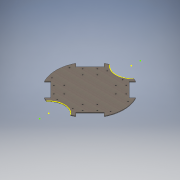
# Autodesk Inventor part: floor_v2
Saved by Autodesk Inventor 2020 (Build 240168000, 168)
## iProperties
Created: 2024-09-07
Part Number: floor_v2
Material: Алюминий 6061
Document SubType Name: Modeling
Designer: Ivan
Density: 2.7 g/cm^3
Appearance: Орех
Mass: 210.887 g
Surface Area: 551.998 cm^2
Volume: 78.1062 cm^3
Author: Ivan
Autodesk Inventor part; units mm, degrees
ref_plane "YZ Plane" through (0, 0, 0) normal (1, 0, 0) x (0, 1, 0)
ref_plane "XZ Plane" through (0, 0, 0) normal (0, 1, 0) x (-1, 0, 0)
ref_plane "XY Plane" through (0, 0, 0) normal (0, 0, 1) x (1, 0, 0)
sketch "Эскиз2" plane through (0, 0, 0) normal (0, 1, 0) x (1, 0, 0)
  circle A0 centre (0, 0) radius 107.5
  circle A1 centre (0, 0) radius 104
  line L0 (0, 0) -> (104, 0) construction
  line L1 (0, 0) -> (0, -104) construction
  line L2 (0, 0) -> (-104, 0) construction
  line L3 (0, 0) -> (0, 104) construction
  line L4 (104, 0) -> (0, -104) construction
  line L5 (0, 104) -> (-104, 0) construction
  line L6 (0, -104) -> (-104, 0) construction
  line L7 (104, 0) -> (0, 104) construction
  line L8 (0, 0) -> (-73.5391, -73.5391) construction
  line L9 (0, 0) -> (73.5391, -73.5391) construction
  line L10 (0, 0) -> (73.5391, 73.5391) construction
  line L11 (0, 0) -> (-73.5391, 73.5391) construction
  line L12 (-38.4471, -82.2877) -> (-82.2877, -38.4471)
  line L13 (-38.4471, -82.2877) -> (-48.2758, -92.1165)
  line L14 (-82.2877, -38.4471) -> (-92.1165, -48.2758)
  line L15 (92.1165, -48.2758) -> (82.2877, -38.4471)
  line L16 (82.2877, -38.4471) -> (38.4471, -82.2877)
  line L17 (38.4471, -82.2877) -> (48.2758, -92.1165)
  line L18 (48.2758, 92.1165) -> (38.4471, 82.2877)
  line L19 (38.4471, 82.2877) -> (82.2877, 38.4471)
  line L20 (82.2877, 38.4471) -> (92.1165, 48.2758)
  line L21 (-48.2758, 92.1165) -> (-38.4471, 82.2877)
  line L22 (-38.4471, 82.2877) -> (-82.2877, 38.4471)
  line L23 (-82.2877, 38.4471) -> (-92.1165, 48.2758)
  line L24 (0, -107.5) -> (0, -79.5) construction
  circle A2 centre (0, -116.5) radius 37 construction
  circle A3 centre (0, -127) radius 47.5
  line L25 (0, 107.5) -> (0, 79.5) construction
  circle A4 centre (0, 127) radius 47.5
  line L26 (-92.1165, 48.2758) -> (-94.7051, 50.8645)
  line L27 (-48.2758, 92.1165) -> (-50.8645, 94.7051)
  line L28 (48.2758, 92.1165) -> (50.8645, 94.7051)
  line L29 (92.1165, 48.2758) -> (94.7051, 50.8645)
  line L30 (92.1165, -48.2758) -> (94.7051, -50.8645)
  line L31 (48.2758, -92.1165) -> (50.8645, -94.7051)
  line L32 (-92.1165, -48.2758) -> (-94.7051, -50.8645)
  line L33 (-48.2758, -92.1165) -> (-50.8645, -94.7051)
  point P0 (-52, -52)
  point P1 (-52, 52)
  point P2 (52, 52)
  point P3 (52, -52)
  point P4 (-60.3674, -60.3674)
  point P5 (60.3674, -60.3674)
  point P6 (60.3674, 60.3674)
  point P7 (-60.3674, 60.3674)
  point P8 (-36.9892, -97.1998)
  point P9 (36.9892, -97.1998)
  point P10 (36.9892, 97.1998)
  point P11 (-36.9892, 97.1998)
  dimension "d137" = 215
  dimension "d138" = 208
  dimension "d143" = 74
  dimension "d144" = 95
  dimension "d140" = 62
  dimension "d141" = 13.9
  dimension "d142" = 28
  constraints: 68 end point, 15 point on line, 14 equal length, 10 perpendicular, 8 collinear, 8 midpoint, 5 parallel, 2 coincident, 2 horizontal, 2 vertical, 1 vertical alignment, 32 other
  measures "d140" distance from line of L14 L12.start
  measures "d141" distance from line of L12 L13.end
  measures "d142" distance of L24.start L24.end
extrude "Выдавливание1" add sketch "Эскиз2" along normal blind 2 contours A1 L15 L16 L17 A3 L13 L12 L14 L23 L22 L21 A4 L18 L19 L20
sketch "Эскиз3" plane through (0, 2, 0) normal (0, -1, 0) x (-1, 0, 0)
  line L0 (33.8509, 77.6915) -> (77.6915, 33.8509) construction
  line L1 (55.7712, 55.7712) -> (0, 0) construction
  line L2 (44.4575, 67.0849) -> (67.0849, 44.4575) construction
  circle A0 centre (44.4575, 67.0849) radius 1.5
  circle A1 centre (67.0849, 44.4575) radius 1.5
  line L3 (28.3991, 51.0265) -> (51.0265, 28.3991) construction
  circle A2 centre (28.3991, 51.0265) radius 1.5
  circle A3 centre (51.0265, 28.3991) radius 1.5
  line L4 (44.4575, -67.0849) -> (67.0849, -44.4575) construction
  line L5 (28.3991, -51.0265) -> (51.0265, -28.3991) construction
  line L6 (55.7712, -55.7712) -> (0, 0) construction
  line L7 (-44.4575, -67.0849) -> (-67.0849, -44.4575) construction
  line L8 (-28.3991, -51.0265) -> (-51.0265, -28.3991) construction
  line L9 (-55.7712, -55.7712) -> (0, 0) construction
  line L10 (-67.0849, 44.4575) -> (-44.4575, 67.0849) construction
  line L11 (-51.0265, 28.3991) -> (-28.3991, 51.0265) construction
  line L12 (-55.7712, 55.7712) -> (0, 0) construction
  circle A4 centre (-44.4575, 67.0849) radius 1.5
  circle A5 centre (-67.0849, 44.4575) radius 1.5
  circle A6 centre (-28.3991, 51.0265) radius 1.5
  circle A7 centre (-51.0265, 28.3991) radius 1.5
  circle A8 centre (-44.4575, -67.0849) radius 1.5
  circle A9 centre (-67.0849, -44.4575) radius 1.5
  circle A10 centre (-51.0265, -28.3991) radius 1.5
  circle A11 centre (-28.3991, -51.0265) radius 1.5
  circle A12 centre (44.4575, -67.0849) radius 1.5
  circle A13 centre (28.3991, -51.0265) radius 1.5
  circle A14 centre (51.0265, -28.3991) radius 1.5
  circle A15 centre (67.0849, -44.4575) radius 1.5
  line L13 (-38.4471, -82.2877) -> (-82.2877, -38.4471) projected
  line L14 (82.2877, -38.4471) -> (38.4471, -82.2877) projected
  line L15 (38.4471, 82.2877) -> (82.2877, 38.4471) projected
  line L16 (-82.2877, 38.4471) -> (-38.4471, 82.2877) projected
  line L17 (82.2877, 38.4471) -> (92.1165, 48.2758) projected
  point P0 (39.7128, 39.7128)
  point P1 (-39.7128, -39.7128)
  point P2 (39.7128, -39.7128)
  point P3 (-39.7128, 39.7128)
  point P4 (-40.1306, -40.1306)
  dimension "d83" = 16
  dimension "d84" = 3
  dimension "d85" = 3
  dimension "d86" = 22.71
  dimension "d87" = 3
  dimension "d88" = 3
  dimension "d89" = 22.71
  dimension "d90" = 22.71
  dimension "d91" = 22.71
  dimension "d95" = 3
  dimension "d96" = 3
  dimension "d97" = 3
  dimension "d98" = 3
  dimension "d99" = 3
  dimension "d100" = 3
  dimension "d101" = 3
  dimension "d102" = 3
  dimension "d103" = 3
  dimension "d104" = 3
  dimension "d105" = 3
  dimension "d106" = 3
  dimension "d145" = 6.5
  dimension "d146" = 6.5
  dimension "d147" = 6.5
  dimension "d148" = 6.5
  constraints: 26 end point, 16 centre point, 16 coincident, 10 point on line, 9 midpoint, 8 equal length, 8 parallel, 2 perpendicular, 1 collinear
  measures "d83" distance from line of L1 L2.start
  measures "d84" diameter of A0
  measures "d85" diameter of A1
  measures "d86" distance from line of L3 L1.start
  measures "d87" diameter of A2
  measures "d88" diameter of A3
  measures "d89" distance from line of L5 L6.start
  measures "d90" distance from line of L11 L12.start
  measures "d91" distance from line of L8 L9.start
  measures "d95" diameter of A4
  measures "d96" diameter of A5
  measures "d97" diameter of A6
  measures "d98" diameter of A7
  measures "d99" diameter of A8
  measures "d100" diameter of A9
  measures "d101" diameter of A10
  measures "d102" diameter of A11
  measures "d103" diameter of A12
  measures "d104" diameter of A13
  measures "d105" diameter of A14
  measures "d106" diameter of A15
  measures "d145" distance from line of L15 L1.start
  measures "d146" distance from line of L16 L12.start
  measures "d147" distance from line of L13 L9.start
  measures "d148" distance from line of L6.start L14
extrude "Выдавливание5" cut sketch "Эскиз3" along normal through all
sketch "Эскиз6" plane through (0, 2, 0) normal (0, -1, 0) x (-1, 0, 0)
  arc A0 (36.9892, -97.1998) -> (-36.9892, -97.1998) centre (0, -127) ccw projected
  arc A1 (-36.9892, 97.1998) -> (36.9892, 97.1998) centre (0, 127) ccw projected
  point P0 (-0.0301, 154.5629)
  point P1 (-0.0412, -154.5628)
sketch "Эскиз7" plane through (0, 2, 0) normal (0, -1, 0) x (-1, 0, 0)
  circle A0 centre (0, 0) radius 94.2655 construction
  circle A1 centre (-90.3481, 26.8924) radius 1.5
  circle A2 centre (-90.3481, -26.8924) radius 1.5
  circle A3 centre (90.3481, 26.8924) radius 1.5
  circle A4 centre (90.3481, -26.8924) radius 1.5
  line L0 (-92.1165, 48.2758) -> (-82.2877, 38.4471) projected
  line L1 (-82.2877, -38.4471) -> (-92.1165, -48.2758) projected
  line L2 (92.1165, -48.2758) -> (82.2877, -38.4471) projected
  line L3 (82.2877, 38.4471) -> (92.1165, 48.2758) projected
  dimension "d119" = 188.531
  dimension "d120" = 3
  dimension "d121" = 3
  dimension "d124" = 3
  dimension "d125" = 3
  dimension "d149" = 13.87
  dimension "d150" = 13.87
  dimension "d151" = 13.87
  dimension "d152" = 13.87
  constraints: 5 centre point, 4 point on circle, 1 coincident
  measures "d119" diameter of A0
  measures "d120" diameter of A1
  measures "d121" diameter of A2
  measures "d124" diameter of A3
  measures "d125" diameter of A4
  measures "d149" distance from line of L0 A1.centre
  measures "d150" distance from line of L1 A2.centre
  measures "d151" distance from line of L2 A4.centre
  measures "d152" distance from line of L3 A3.centre
extrude "Выдавливание4" cut sketch "Эскиз7" along normal through all
sketch "Эскиз8" plane through (0, 2, 0) normal (0, 1, 0) x (1, 0, 0)
  arc A0 (-48.2758, -92.1165) -> (-36.9892, -97.1998) centre (0, 0) ccw projected
  arc A1 (36.9892, -97.1998) -> (48.2758, -92.1165) centre (0, 0) ccw projected
  arc A2 (36.9892, -97.1998) -> (-36.9892, -97.1998) centre (0, -127) ccw projected
  circle A3 centre (0, -127) radius 55.4164 construction
  circle A4 centre (-23.8556, -76.9811) radius 1.5
  circle A5 centre (23.8556, -76.9811) radius 1.5
  circle A6 centre (-28.3991, -51.0265) radius 1.5 construction
  circle A7 centre (-51.0265, -28.3991) radius 1.5 construction
  circle A8 centre (-67.0849, -44.4575) radius 1.5 construction
  circle A9 centre (-44.4575, -67.0849) radius 1.5 construction
  circle A10 centre (-51.0265, -28.3991) radius 1.5 construction
  line L0 (-51.0265, -28.3991) -> (-28.3991, -51.0265) construction
  line L1 (-67.0849, -44.4575) -> (-44.4575, -67.0849) construction
  line L2 (-55.7712, -55.7712) -> (-39.7128, -39.7128) construction
  line L3 (-50.4184, -50.4184) -> (-23.8556, -76.9811) construction
  circle A11 centre (67.0849, -44.4575) radius 1.5 construction
  circle A12 centre (44.4575, -67.0849) radius 1.5 construction
  line L4 (44.4575, -67.0849) -> (67.0849, -44.4575) construction
  arc A13 (-92.1165, 48.2758) -> (-92.1165, -48.2758) centre (0, 0) ccw construction
  line L5 (-104, 0) -> (104, 0) construction
  arc A14 (92.1165, -48.2758) -> (92.1165, 48.2758) centre (0, 0) ccw construction
  circle A15 centre (-23.8556, 76.9811) radius 1.5
  circle A16 centre (23.8556, 76.9811) radius 1.5
  point P0 (-44.5136, -93.9922)
  point P1 (-104, 0)
  dimension "d153" = 11.2867
  dimension "d154" = 3.7622
  dimension "d156" = 22.71
  dimension "d157" = 7.57
  dimension "d158" = 7.57
  constraints: 12 end point, 7 point on circle, 5 centre point, 2 equal radius, 2 midpoint, 2 symmetric about line, 1 coincident, 1 horizontal, 1 perpendicular, 1 point on line, 2 other
  measures "d153" horizontal distance of A0.end A0.start
  measures "d154" horizontal distance of A3.start A0.start
  measures "d156" distance from line of L0 L2.start
  measures "d157" distance from line of L1 L3.start
  measures "d158" distance from line of L4 A5.centre
extrude "Выдавливание6" cut sketch "Эскиз8" against normal through all
equation "\"d85\" = d84"
equation "\"d87\" = d84"
equation "\"d88\" = d84"
